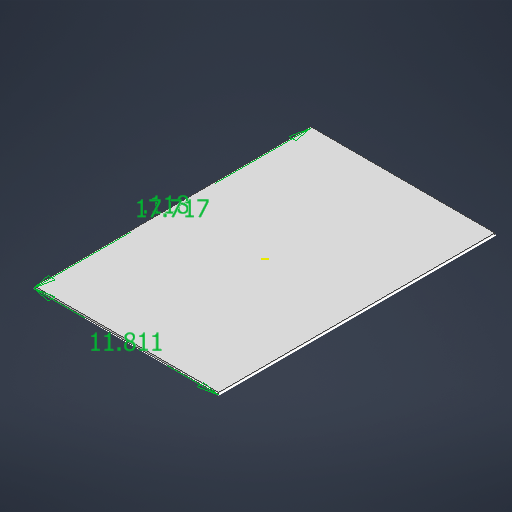
# Autodesk Inventor part: Part2
Saved by Autodesk Inventor 2026.2 (Build 302298010, 298A)
## iProperties
Created: 2026-03-25
Part Number: Part2
Material: Generic
Document SubType Name: Modeling
Designer: Srishanth Dhondy
Density: 1 g/cm^3
Appearance: Default
Author: Srishanth Dhondy
Autodesk Inventor part; units mm, degrees
ref_plane "YZ Plane" through (0, 0, 0) normal (1, 0, 0) x (0, 1, 0)
ref_plane "XZ Plane" through (0, 0, 0) normal (0, 1, 0) x (-1, 0, 0)
ref_plane "XY Plane" through (0, 0, 0) normal (0, 0, 1) x (1, 0, 0)
sketch "Sketch1" plane through (0, 0, 0) normal (0, 1, 0) x (-1, 0, 0)
  line L0 (-150, -225) -> (150, -225)
  line L1 (150, -225) -> (150, 225)
  line L2 (150, 225) -> (-150, 225)
  line L3 (-150, 225) -> (-150, -225)
  line L4 (-150, -225) -> (150, 225) construction
  line L5 (150, -225) -> (-150, 225) construction
  line L6 (147, 222) -> (147, -222)
  line L7 (147, -222) -> (-147, -222)
  line L8 (-147, -222) -> (-147, 222)
  line L9 (-147, 222) -> (147, 222)
  point P0 (0, 0)
  dimension "d0" = 300
  dimension "d1" = 450
  dimension "d4" = 3
  constraints: 20 end point, 4 parallel, 2 midpoint, 2 perpendicular, 1 horizontal, 3 other
  measures "d0" distance of L2.end L1.end
  measures "d1" distance of L1.end L0.end
  measures "d4" distance between parallel lines of L1 L6
extrude "Extrusion1" add sketch "Sketch1" along normal blind 3 contours L3 L2 L1 L0 | L6 L7 L8 L9
body "Solid1"
